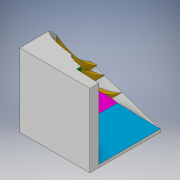
# Autodesk Inventor part: Part1
Saved by Autodesk Inventor 2019.3 (Build 233278000, 278)
## iProperties
Created: 2019-09-21
Part Number: Part1
Material: Generic
Document SubType Name: Modeling
Designer: dell
Density: 1 g/cm^3
Appearance: Default
Author: dell
Autodesk Inventor part; units mm, degrees
sketch "Sketch1" plane through (0, 0, 0) normal (0, 1, 0) x (-1, 0, 0)
  line L0 (0, 0) -> (120, 0)
  line L1 (120, 0) -> (120, -50)
  line L2 (0, 0) -> (0, -15)
  line L3 (40, -25) -> (40, -17)
  line L4 (40, -17) -> (0, -15)
  line L5 (120, -50) -> (120, -120)
  line L6 (120, -120) -> (0, -120)
  line L7 (0, -120) -> (0, -15)
  line L8 (40, -25) -> (62.7504, -27.9567) construction
  line L9 (62.7504, -27.9567) -> (65.3277, -34.1422) construction
  spline S0 degree 2 poles (40, -25) (62.7504, -27.9567) (65.3277, -34.1422) knots 1 1 1 2 2 2
  line L10 (65.3277, -34.1422) -> (111.1336, -40.0952) construction
  line L11 (111.1336, -40.0952) -> (120, -50) construction
  spline S1 degree 2 poles (65.3277, -34.1422) (111.1336, -40.0952) (120, -50) knots 1 1 1 2 2 2
  line L12 (0, -15) -> (0, -120)
  line L13 (10.0304, -120) -> (10.0304, -15)
  line L14 (10.0304, -15) -> (0, -15)
  dimension "d0" = 120
  dimension "d1" = 50
  dimension "d2" = 15
  dimension "d5" = 8
  dimension "d7" = 70
  constraints: 22 end point, 4 vertical, 2 collinear, 2 horizontal, 1 parallel, 1 perpendicular, 1 point on line, 6 other
  measures "d0" distance of L0.start L0.end
  measures "d1" distance of L0.end L1.end
  measures "d2" distance of L0.start L2.end
  measures "d5" distance of L3.start L3.end
  measures "d7" distance of L1.end L5.end
ref_plane "Work Plane2" through (-120, 0, -120) normal (0, 0, 1) x (1, 0, 0)
sketch "Sketch2" plane through (-120, 0, -120) normal (0, 0, 1) x (1, 0, 0)
  line L0 (80, 0) -> (0, 0) projected
  line L1 (0, 0) -> (0, 40)
  line L2 (0, 0) -> (0, 120) projected
  line L3 (120, 0) -> (0, 40)
  line L4 (0, 40) -> (0, 0)
  line L5 (120, 0) -> (80, 0) projected
  line L6 (0, 0) -> (120, 0)
  line L7 (0, 0) -> (0, 35)
  line L8 (0, 35) -> (15, 35)
  dimension "d12" = 40
  dimension "d20" = 35
  constraints: 12 end point, 3 point on line, 2 collinear, 1 perpendicular
  measures "d12" distance of L0.end L1.end
  measures "d20" distance of L0.end L7.end
extrude "Extrusion2" add sketch "Sketch1" along normal blind 120 contours L0 L1 S1 S0 L3 L4 L13 L14 L2 | L14 L13 L4
extrude "Extrusion3" add sketch "Sketch2" along normal blind 120
ref_plane "Work Plane4" through (-120, 0, 0) normal (-1, 0, 0) x (0, 0, 1)
ref_plane "Work Plane3" through (-65.24, 0, 0) normal (-1, 0, 0) x (0, 0, 1)
ref_plane "Work Plane5" through (0, 35, 0) normal (0, -1, 0) x (1, 0, 0)
sketch "Sketch3" plane through (0, 35, 0) normal (0, -1, 0) x (1, 0, 0)
  line L0 (-40, -17) -> (-40, -25) projected
  line L1 (-40, -25) -> (-40, -120)
  line L2 (-120, -120) -> (0, -120) projected
  line L3 (-40, -120) -> (-65.3277, -120)
  line L4 (-65.3277, -120) -> (-65.3277, -34.1422)
  line L5 (-65.3277, -34.1422) -> (-40, -25)
  point P0 (0, 0)
  constraints: 8 end point, 2 point on line, 2 vertical
ref_plane "Work Plane6" through (-40, 35, -25) normal (-0.6585046, -0.7525767, 0) x (0, 0, -1)
sketch "Sketch4" plane through (-40, 35, -25) normal (-0.6585046, -0.7525767, 0) x (0, 0, -1)
  line L0 (-8, 14.2676) -> (-8, -55.9729) projected
  line L1 (-8, -0.0285) -> (-10.0799, 53.1079)
  line L2 (-8, -0.0285) -> (62, 0)
  line L3 (0, 0) -> (95, 0) projected
  line L4 (95, 53.1507) -> (95, -63.4987) projected
  line L5 (62, 0) -> (95, 53.1507)
  line L6 (95, 53.1507) -> (-10.0799, 53.1079)
  point P0 (-25, 53.1507)
  dimension "d23" = 70
  constraints: 8 end point, 2 point on line, 1 parallel
  measures "d23" distance of L1.start L2.end
extrude "Extrusion5" add sketch "Sketch4" along normal blind 3 contours L1 L6 L5 L2
ref_plane "Work Plane7" through (0, 60, 0) normal (0, -1, 0) x (1, 0, 0)
sketch "Sketch5" plane through (0, 60, 0) normal (0, -1, 0) x (1, 0, 0)
  line L0 (-65.3277, -34.1422) -> (-65.3277, -119.3385)
  line L1 (-65.3277, -119.3385) -> (-65.3277, -54.3385)
  line L2 (-65.3277, -54.3385) -> (-74.8086, -54.3385)
  point P0 (0, 0)
  dimension "d27" = 65
  constraints: 6 end point, 1 perpendicular, 1 point on line, 1 vertical
  measures "d27" distance of L0.end L1.end
ref_plane "Work Plane8" through (-65.3277, 60, -34.1422) normal (-0.7024879, -0.7116957, 0) x (0, 0, -1)
sketch "Sketch6" plane through (-65.3277, 60, -34.1422) normal (-0.7024879, -0.7116957, 0) x (0, 0, -1)
  line L0 (-9.1422, 35.5878) -> (-9.1422, -24.1237) projected
  line L1 (-9.1422, 35.5878) -> (3.8699, 3.2623) construction
  line L2 (3.8699, 3.2623) -> (20.2466, 0.13) construction
  line L3 (20.2466, 0.13) -> (20.3011, 0.13) construction
  spline S0 degree 3 poles (-9.1422, 35.5878) (3.8699, 3.2623) (20.2466, 0.13) (20.3011, 0.13) knots 1 1 1 1 2 2 2 2
  line L4 (52.8578, 35.5878) -> (85.8578, 88.6427) projected
  line L5 (52.8578, 35.5878) -> (39.1413, 5.7321) construction
  line L6 (39.1413, 5.7321) -> (20.3011, 0.13) construction
  spline S1 degree 2 poles (52.8578, 35.5878) (39.1413, 5.7321) (20.3011, 0.13) knots 1 1 1 2 2 2
  line L7 (52.8578, 35.5878) -> (-9.1422, 35.5878)
  point P0 (-34.1422, 88.6427)
  constraints: 2 end point, 2 horizontal, 6 other
extrude "Extrusion6" add sketch "Sketch6" along normal blind 10
sketch "Sketch7" plane through (-120, 0, 0) normal (-1, 0, 0) x (0, 0, 1)
  line L0 (-50, 120) -> (0, 120) projected
  line L1 (-50, 120) -> (-125, 120)
  line L2 (-125, 120) -> (-125, 39.626)
  line L3 (-125, 39.626) -> (-50, 39.626)
  line L4 (-50, 39.626) -> (-50, 120)
  point P0 (0, 0)
  dimension "d30" = 75
  constraints: 8 end point, 2 horizontal, 2 perpendicular
  measures "d30" distance of L0.start L1.end
ref_plane "Work Plane11" through (-65, 0, 0) normal (-1, 0, 0) x (0, 0, 1)
ref_plane "Work Plane12" through (-40, 13.3333, -17) normal (0.3162278, 0.9486833, 0) x (0.9486833, -0.3162278, 0)
sketch "Sketch12" plane through (-40, 13.3333, -17) normal (0.3162278, 0.9486833, 0) x (0.9486833, -0.3162278, 0)
  point P0 (42.1637, -17)
ref_plane "Work Plane13" through (-120, 40, -120) normal (-0.9486833, 0.3162278, 0) x (0, 0, 1)
sketch "Sketch13" plane through (-120, 40, -120) normal (-0.9486833, 0.3162278, 0) x (0, 0, 1)
  line L0 (0, 0) -> (0, -37.9473) projected
  line L1 (81.226, 84.3255) -> (81.226, -3.4229)
  line L2 (81.226, -3.4229) -> (0, -0.3549)
  line L3 (81.226, 84.3255) -> (95, 183.3723)
  line L4 (0, 0) -> (70, 0) projected
  line L5 (0, 0) -> (-100, 0)
  point P0 (120, 0)
  dimension "d37" = 100
  dimension "d38" = 100
  constraints: 8 end point, 1 horizontal, 1 vertical
  measures "d37" distance of L1.start L3.end
  measures "d38" distance of L0.start L5.end
ref_plane "Work Plane14" through (-77.831, 25.9437, -120) normal (-0.9486833, 0.3162278, 0) x (0, 0, 1)
ref_plane "Work Plane16" through (-65.5, 0, 0) normal (-1, 0, 0) x (0, 0, 1)
sketch "Sketch17" plane through (-40, 13.3333, -17) normal (0.3162278, 0.9486833, 0) x (0.9486833, -0.3162278, 0)
  line L0 (-26.635, 17.3556) -> (-26.635, 102.3556)
  line L1 (42.1637, 103) -> (-84.3274, 103) projected
  line L2 (-26.635, 17.3556) -> (58.365, 17.3556) construction
  point P0 (42.1637, -17)
  point P1 (-26.635, 103)
  dimension "d46" = 85
  dimension "d47" = 90
  constraints: 4 end point, 2 perpendicular, 1 horizontal
  measures "d46" distance of L0.start L0.end
  measures "d47" angle of L2 L0
ref_plane "Work Plane18" through (-65, 0, 0) normal (-1, 0, 0) x (0, 0, 1)
sketch "Sketch18" plane through (-65, 0, 0) normal (-1, 0, 0) x (0, 0, 1)
  spline S0 degree 2 poles (-34.1422, 120) (-48.3232, 65.055) (-54.4434, 59.9087) knots 1 1 1 2 2 2 projected
  line L0 (-34.1422, 21.7759) -> (-34.1422, 120) projected
  line L1 (-120, 39.626) -> (-120, 0) projected
  line L2 (-120, 21.7759) -> (-64.343, 52.126) construction
  line L3 (-64.343, 52.126) -> (-54.4434, 59.9087) construction
  spline S1 degree 2 poles (-120, 21.7759) (-64.343, 52.126) (-54.4434, 59.9087) knots 1 1 1 2 2 2
  line L4 (-34.1422, 21.7759) -> (-34.1422, 120) projected
  line L5 (-34.1422, 21.7759) -> (-120, 21.7759)
  line L6 (-120, 21.7759) -> (-34.1422, 21.7759)
  point P0 (0, 0)
  constraints: 4 end point, 1 collinear, 1 perpendicular, 1 point on line, 3 other
ref_plane "Work Plane19" through (-95, 0, 0) normal (-1, 0, 0) x (0, 0, 1)
sketch "Sketch19" plane through (-95, 0, 0) normal (-1, 0, 0) x (0, 0, 1)
  line L0 (-39.2565, 119.979) -> (-79.1624, 47.7695) construction
  line L1 (-79.1624, 47.7695) -> (-119.9333, 31.7447) construction
  spline S0 degree 2 poles (-39.2565, 119.979) (-79.1624, 47.7695) (-119.9333, 31.7447) knots 1 1 1 2 2 2
  line L2 (-119.9333, 31.7447) -> (-39.2565, 31.7447)
  line L3 (-39.2565, 31.7447) -> (-39.2565, 119.979)
  point P0 (0, 0)
  constraints: 4 end point, 1 horizontal, 1 perpendicular, 3 other
extrude "Extrusion11" add sketch "Sketch19" along normal blind 25
ref_plane "Work Plane20" through (-120, 20, -120) normal (-1, 0, 0) x (0, 0, 1)
sketch "Sketch20" plane through (-120, 20, -120) normal (-1, 0, 0) x (0, 0, 1)
  line L0 (70, 19.813) -> (70, 100.187) projected
  line L1 (70, 100.187) -> (32.2352, 35.2872) construction
  line L2 (0, 20.187) -> (15.7371, 20.187) projected
  line L3 (32.2352, 35.2872) -> (0, 20.187) construction
  spline S0 degree 2 poles (70, 100.187) (32.2352, 35.2872) (0, 20.187) knots 1 1 1 2 2 2
  line L4 (70, 19.813) -> (70, 81.7691) projected
  line L5 (70, 100.187) -> (70, 19.813)
  line L6 (70, 19.813) -> (0, 20.187)
  point P0 (120, -20)
  constraints: 4 end point, 1 vertical, 3 other
extrude "Extrusion12" add sketch "Sketch20" against normal blind 12.5
ref_plane "Work Plane21" through (-65, 0, 0) normal (-1, 0, 0) x (0, 0, 1)
sketch "Sketch21" plane through (-65, 0, 0) normal (-1, 0, 0) x (0, 0, 1)
  line L0 (-54.4434, 59.9087) -> (-54.4434, 52.7917) projected
  line L1 (-54.4434, 59.9087) -> (-101.2792, 22.7184) construction
  line L2 (-101.2792, 22.7184) -> (-120, 21.6563) construction
  spline S0 degree 2 poles (-54.4434, 59.9087) (-101.2792, 22.7184) (-120, 21.6563) knots 1 1 1 2 2 2
  line L3 (-120, 21.6563) -> (-34.1422, 21.6563)
  line L4 (-34.1422, 21.7759) -> (-34.1422, 120) projected
  line L5 (-34.1422, 21.6563) -> (-34.1422, 120)
  line L6 (-34.1422, 120) -> (-34.1422, 21.6563)
  line L7 (-34.1422, 120) -> (-44.5669, 67.7512) construction
  line L8 (-44.5669, 67.7512) -> (-54.4434, 59.9087) construction
  spline S1 degree 2 poles (-34.1422, 120) (-44.5669, 67.7512) (-54.4434, 59.9087) knots 1 1 1 2 2 2
  point P0 (0, 0)
  constraints: 6 end point, 1 collinear, 1 horizontal, 1 perpendicular, 6 other
extrude "Extrusion13" add sketch "Sketch21" along normal blind 40
extrude "Extrusion14" add sketch "Sketch1" against normal blind 5
body "Solid2"
